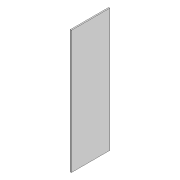
# Autodesk Inventor part: LR_Sides
Saved by Autodesk Inventor 2021.3 (Build 253353000, 353)
## iProperties
Created: 2021-11-26
Part Number: LR_Sides
Material: Generic
Document SubType Name: Modeling
Designer: wbrooks
Density: 1 g/cm^3
Appearance: Default
Author: wbrooks
Autodesk Inventor part; units mm, degrees
ref_plane "YZ Plane" through (0, 0, 0) normal (1, 0, 0) x (0, 1, 0)
ref_plane "XZ Plane" through (0, 0, 0) normal (0, 1, 0) x (-1, 0, 0)
ref_plane "XY Plane" through (0, 0, 0) normal (0, 0, 1) x (1, 0, 0)
sketch "Sketch1" plane through (0, 0, 0) normal (1, 0, 0) x (0, 1, 0)
  line L0 (609.6, -189.7062) -> (-609.6, -189.7063)
  line L1 (-609.6, -189.7063) -> (-609.6, 189.7062)
  line L2 (-609.6, 189.7062) -> (609.6, 189.7063)
  line L3 (609.6, 189.7063) -> (609.6, -189.7062)
  line L4 (609.6, -189.7062) -> (-609.6, 189.7062) construction
  line L5 (-609.6, -189.7063) -> (609.6, 189.7063) construction
  point P0 (0, 0)
  dimension "d2" = 1219.2
  dimension "d3" = 379.4125
  constraints: 12 end point, 2 midpoint, 2 parallel, 1 horizontal, 1 perpendicular
  measures "d2" distance of L1.end L2.end
  measures "d3" distance of L0.end L1.end
extrude "Extrusion1" add sketch "Sketch1" along normal mid plane 11.9062
body "Solid1"
